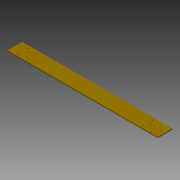
# Autodesk Inventor part: X Rail
Saved by Autodesk Inventor 2013 SP2 (Build 170200200, 200)
## iProperties
Created: 2017-01-25
Part Number: X Rail
Material: Generic
Document SubType Name: Modeling
Designer: Herman de Vries
Density: 1 g/cm^3
Mass: 71.8002 g
Surface Area: 513.07 cm^2
Volume: 71.8002 cm^3
Author: Herman de Vries
Autodesk Inventor part; units mm, degrees
ref_plane "YZ Plane" through (0, 0, 0) normal (1, 0, 0) x (0, 1, 0)
ref_plane "XZ Plane" through (0, 0, 0) normal (0, 1, 0) x (-1, 0, 0)
ref_plane "XY Plane" through (0, 0, 0) normal (0, 0, 1) x (1, 0, 0)
sketch "Sketch1" plane through (0, 0, 0) normal (1, 0, 0) x (0, 1, 0)
  line L0 (0, 0) -> (50, 0)
  line L1 (50, 0) -> (50, 3)
  line L2 (50, 3) -> (0, 3)
  line L3 (0, 3) -> (0, 0)
  dimension "d0" = 50
  dimension "d1" = 3
  constraints: 8 end point, 2 parallel, 1 horizontal, 1 perpendicular
  measures "d0" distance of L2.end L1.end
  measures "d1" distance of L1.end L0.end
extrude "Extrusion1" add sketch "Sketch1" along normal blind 510
sketch "Sketch2" plane through (0, 0, 3) normal (0, 0, 1) x (1, 0, 0)
  line L0 (0, 0) -> (510, 0) projected
  line L1 (0, 50) -> (510, 50) projected
  line L2 (0, 50) -> (0, 0) projected
  line L3 (510, 50) -> (510, 0) projected
  line L4 (30, 9.5) -> (61, 9.5) construction
  line L5 (61, 9.5) -> (61, 40.5) construction
  line L6 (61, 40.5) -> (30, 40.5) construction
  line L7 (30, 40.5) -> (30, 9.5) construction
  circle A0 centre (30, 40.5) radius 1.5
  circle A1 centre (61, 40.5) radius 1.5
  circle A2 centre (61, 9.5) radius 1.5
  circle A3 centre (30, 9.5) radius 1.5
  circle A4 centre (500, 23) radius 1.5
  circle A5 centre (472, 13) radius 1.6 projected
  circle A6 centre (458, 27) radius 1.6 projected
  circle A7 centre (451, 40.5) radius 1.65 projected
  circle A8 centre (451, 9.5) radius 1.65 projected
  circle A9 centre (52, 13) radius 1.6 projected
  circle A10 centre (38, 27) radius 1.6 projected
  circle A11 centre (483, 36) radius 1.6 projected
  circle A12 centre (483, 4) radius 1.6 projected
  circle A13 centre (7, 36) radius 1.6 projected
  circle A14 centre (7, 4) radius 1.6 projected
  point P0 (30, 25)
  point P1 (510, 25)
  dimension "d12" = 31
  dimension "d13" = 31
  dimension "d14" = 30
  dimension "d15" = 3
  dimension "d16" = 3
  dimension "d17" = 3
  dimension "d18" = 3
  dimension "d26" = 3
  dimension "d27" = 10
  dimension "d35" = 23
  constraints: 8 end point, 5 centre point, 4 coincident, 2 midpoint, 2 parallel, 1 horizontal, 1 perpendicular
  measures "d12" distance of L6.end L5.end
  measures "d13" distance of L5.end L4.end
  measures "d14" distance between parallel lines of L2 L7
  measures "d15" diameter of A0
  measures "d16" diameter of A1
  measures "d17" diameter of A2
  measures "d18" diameter of A3
  measures "d26" diameter of A4
  measures "d27" distance from line of A4.centre L3
  measures "d35" distance from line of L0 A4.centre
extrude "Extrusion2" cut sketch "Sketch2" against normal blind 10 contours A0 | A1 | A2 | A3 | A4 | A5 | A6 | A7 | A8 | A9 | A10 | A11 | A12 | A13 | A14
equation "\"d12\" = d13"
body "Solid1"
